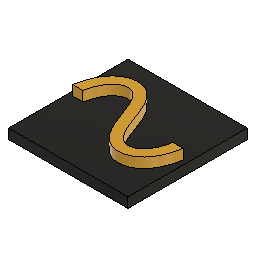
icon_system (Autodesk Fusion 360 design; units mm, degrees)
Autodesk Fusion 360 part; units mm, degrees
sketch "Sketch1" plane through (0, 0, 0) normal (0, 0, 1) x (1, 0, 0)
  line L0 (5.95, -5.95) -> (-5.95, -5.95)
  line L1 (-5.95, -5.95) -> (-5.95, 5.95)
  line L2 (-5.95, 5.95) -> (5.95, 5.95)
  line L3 (5.95, 5.95) -> (5.95, -5.95)
  line L4 (5.95, -5.95) -> (-5.95, 5.95) construction
  line L5 (-5.95, -5.95) -> (5.95, 5.95) construction
  spline S0 degree 5 poles (-5, 0) (-4.9575, 0.2297) (-4.8598, 0.6679) (-4.6747, 1.2621) (-4.3511, 1.9274) (-3.8228, 2.5423) (-3.1921, 2.9282) (-2.4956, 3.0695) (-1.817, 2.932) (-1.2301, 2.5035) (-0.7463, 1.8241) (-0.3498, 0.9601) (-0.0005, -0.0002) (0.351, -0.9598) (0.7529, -1.8223) (1.2432, -2.5008) (1.8348, -2.9297) (2.5144, -3.0694) (3.2094, -2.9308) (3.8371, -2.5468) (4.3614, -1.9323) (4.6812, -1.266) (4.8631, -0.6702) (4.9587, -0.2305) (5, 0) knots 0 0 0 0 0 0 0.05 0.1 0.15 0.2 0.25 0.3 0.35 0.4 0.45 0.5 0.55 0.6 0.65 0.7 0.75 0.8 0.85 0.9 0.95 1 1 1 1 1 1
  line L6 (-3.5, 3) -> (-1.5, 3)
  line L7 (1.5241, -3) -> (3.5241, -3)
  line L8 (-4.4909, 0) -> (-5.55, 0)
  line L9 (4.4915, 0) -> (5.508, 0)
  spline S1 degree 3 poles (-4.4909, 0) (-4.202, 1.4563) (-3.5685, 2.2271) (-2.8864, 2.4394) (-2.3165, 2.6168) (-1.8076, 2.4436) (-1.3375, 1.7472) (-0.8557, 1.0334) (-0.503, -0.2172) (-0.0186, -1.3122) (0.3354, -2.1125) (0.7938, -2.8423) (1.4733, -3.2241) (2.1901, -3.6268) (3.0825, -3.561) (3.7767, -3.1336) (4.612, -2.6193) (5.1673, -1.6393) (5.4409, -0.3504) (5.4591, -0.2645) (5.4762, -0.1772) (5.4921, -0.0883) (5.4974, -0.0588) (5.5027, -0.0294) (5.508, 0) knots 0.004254 0.004254 0.004254 0.004254 0.210613 0.210613 0.210613 0.38303 0.38303 0.38303 0.559752 0.559752 0.559752 0.688923 0.688923 0.688923 0.82516 0.82516 0.82516 0.989082 0.989082 0.989082 1 1 1 1.008967 1.008967 1.008967 1.008967
  spline S2 degree 3 poles (-5.5085, 0) (-5.5029, 0.0303) (-5.4973, 0.0606) (-5.4917, 0.0909) (-5.2527, 1.3828) (-4.7611, 2.3804) (-3.9943, 2.9693) (-3.3458, 3.4673) (-2.49, 3.6492) (-1.7382, 3.359) (-1.0443, 3.0912) (-0.5365, 2.4519) (-0.1666, 1.7152) (0.3056, 0.7749) (0.6186, -0.3569) (1.0231, -1.1811) (1.3551, -1.8577) (1.7348, -2.2795) (2.1216, -2.4267) (2.7975, -2.684) (3.6536, -2.3065) (4.1588, -1.1313) (4.2954, -0.8137) (4.4079, -0.4363) (4.4915, 0) knots 0 0 0 0 0.009248 0.009248 0.009248 0.168421 0.168421 0.168421 0.30303 0.30303 0.30303 0.427287 0.427287 0.427287 0.585905 0.585905 0.585905 0.716109 0.716109 0.716109 0.943637 0.943637 0.943637 1.005138 1.005138 1.005138 1.005138
  point P0 (-2.5, 3)
  point P1 (2.5241, -3)
  point P2 (5.4921, -0.0883)
  dimension "d1" = 11.9
  dimension "d2" = 11.9
  constraint horizontal L0
  constraint perpendicular L0 L1
  constraint parallel L0 L2
  constraint parallel L1 L3
  constraint coincident L4 origin
  constraint coincident L5 origin
  constraint midpoint P0 L6
  constraint midpoint P1 L7
  constraint horizontal L8
  constraint coincident L8 S2.start
  constraint horizontal L9
  measures "d1" distance of L1.end L2.end
  measures "d2" distance of L0.end L1.end
extrude "Extrude1" add sketch "Sketch1" against normal blind 1 contours L0 L1 L2 L3 | S0 L8 L9 S2 | S0 L8 L9 S1
extrude "Extrude3" add sketch "Sketch1" along normal blind 1 contours S0 L8 L9 S2 | S0 L8 L9 S1
